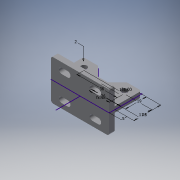
# Autodesk Inventor part: basepart
Saved by Autodesk Inventor 2018 (Build 220112000, 112)
## iProperties
Created: 2018-12-04
Part Number: basepart
Material: Generic
Document SubType Name: Modeling
Designer: Jerry
Density: 1 g/cm^3
Appearance: Default
Author: Jerry
Autodesk Inventor part; units mm, degrees
ref_plane "YZ Plane" through (0, 0, 0) normal (1, 0, 0) x (0, 1, 0)
ref_plane "XZ Plane" through (0, 0, 0) normal (0, 1, 0) x (-1, 0, 0)
ref_plane "XY Plane" through (0, 0, 0) normal (0, 0, 1) x (1, 0, 0)
sketch "Sketch1" plane through (0, 0, 0) normal (0, 0, 1) x (1, 0, 0)
  line L0 (0, 0) -> (0, -31.9527)
  line L1 (13.6569, 19) -> (24, 19)
  line L2 (1.4142, 7.5858) -> (12.2426, 18.4142)
  line L3 (26, 17) -> (26, -10)
  line L4 (26, -10) -> (0, -10)
  line L5 (-13.6569, 19) -> (-24, 19)
  line L6 (-1.4142, 7.5858) -> (-12.2426, 18.4142)
  line L7 (-26, 17) -> (-26, -10)
  line L8 (-26, -10) -> (0, -10)
  line L9 (-26, -5) -> (26, -5)
  arc A0 (-24, 19) -> (-26, 17) centre (-24, 17) ccw
  arc A1 (-12.2426, 18.4142) -> (-13.6569, 19) centre (-13.6569, 17) ccw
  arc A2 (-1.4142, 7.5858) -> (1.4142, 7.5858) centre (0, 9) ccw
  arc A3 (13.6569, 19) -> (12.2426, 18.4142) centre (13.6569, 17) ccw
  arc A4 (26, 17) -> (24, 19) centre (24, 17) ccw
  point P0 (-18, 11.5)
  point P1 (18, 11.5)
  point P2 (12.8284, 19)
  point P3 (26, 19)
  point P4 (-12.8284, 19)
  point P5 (-26, 19)
  dimension "d0" = 36
  dimension "d1" = 18
  dimension "d2" = 135
  dimension "d3" = 19
  dimension "d4" = 11.5
  dimension "d5" = 5
  dimension "d6" = 24
  dimension "d7" = 26
  dimension "d10" = 2
  dimension "d11" = 10
  constraints: 20 end point, 11 point on line, 10 point on circle, 10 tangent, 5 centre point, 4 equal radius, 3 symmetric about line, 2 perpendicular, 2 vertical, 1 horizontal, 1 horizontal alignment, 1 vertical alignment
  measures "d0" distance of point (-18, 11.5) point (18, 11.5)
  measures "d1" horizontal distance of L0.start point (18, 11.5)
  measures "d2" angle of L1 L2
  measures "d3" distance from line of L0.start L1
  measures "d4" vertical distance of L0.start point (-18, 11.5)
  measures "d5" distance between parallel lines of L4 L9
  measures "d6" distance between parallel lines of L1 L9
  measures "d7" distance from line of L0.start L3
  measures "d10" radius of A0
  measures "d11" distance from line of L1 A2.centre
extrude "Extrusion1" add sketch "Sketch1" along normal mid plane 5 contours L9 L7 A0 L5 A1 L6 A2 L2 A3 L1 A4 L3
hole "Hole1" at (-18, 11.5, 0) at (18, 11.5, 0) direction (0, 0, -1) diameter 5.159 end through all both
extrude "Extrusion2" add sketch "Sketch1" along normal mid plane 36 contours L9 L3 L4 L0 | L0 L8 L7 L9
fillet "Fillet1" radius 2 4 edges at (-26, -7.5, 18) (26, -7.5, 18) (-26, -7.5, -18) (26, -7.5, -18)
sketch "Sketch2" plane through (-26, -5, -2.5) normal (0, 1, 0) x (1, 0, 0)
  line L0 (42.418, 8.7532) -> (37.087, 8.7532) construction
  line L1 (42.418, 11.2532) -> (37.087, 11.2532)
  line L2 (37.087, 6.2532) -> (42.418, 6.2532)
  arc A0 (42.418, 6.2532) -> (42.418, 11.2532) centre (42.418, 8.7532) ccw
  arc A1 (37.087, 11.2532) -> (37.087, 6.2532) centre (37.087, 8.7532) ccw
  line L3 (69.9256, -2.5) -> (59.9264, -2.5) projected
  line L4 (36.6897, -2.5) -> (64.1036, -2.5) projected
  line L5 (42.418, -13.7532) -> (37.087, -13.7532) construction
  line L6 (42.418, -16.2532) -> (37.087, -16.2532)
  line L7 (37.087, -11.2532) -> (42.418, -11.2532)
  arc A2 (42.418, -16.2532) -> (42.418, -11.2532) centre (42.418, -13.7532) ccw
  arc A3 (37.087, -11.2532) -> (37.087, -16.2532) centre (37.087, -13.7532) ccw
  line L8 (52, 0) -> (0, 0) projected
  line L9 (26, 0) -> (26, 17.4848)
  line L10 (9.582, 8.7532) -> (14.913, 8.7532) construction
  line L11 (9.582, 11.2532) -> (14.913, 11.2532)
  line L12 (14.913, 6.2532) -> (9.582, 6.2532)
  arc A4 (9.582, 11.2532) -> (9.582, 6.2532) centre (9.582, 8.7532) ccw
  arc A5 (14.913, 6.2532) -> (14.913, 11.2532) centre (14.913, 8.7532) ccw
  line L13 (9.582, -13.7532) -> (14.913, -13.7532) construction
  line L14 (9.582, -16.2532) -> (14.913, -16.2532)
  line L15 (14.913, -11.2532) -> (9.582, -11.2532)
  arc A6 (9.582, -11.2532) -> (9.582, -16.2532) centre (9.582, -13.7532) ccw
  arc A7 (14.913, -16.2532) -> (14.913, -11.2532) centre (14.913, -13.7532) ccw
  point P0 (26, -2.5)
  point P1 (39.7525, 8.7532)
  point P2 (39.7525, -13.7532)
  point P3 (26, -2.5)
  point P4 (26, -2.5)
  point P5 (26, -2.5)
  point P6 (12.2475, 8.7532)
  point P7 (15.3103, -2.5)
  point P8 (12.2475, -13.7532)
  dimension "d24" = 5
  constraints: 34 end point, 22 symmetric about line, 16 point on circle, 8 centre point, 4 tangent, 2 midpoint, 1 horizontal, 1 parallel, 1 vertical, 6 other
  measures "d24" diameter of A1
extrude "Extrusion3" cut sketch "Sketch2" against normal through all
equation "\"d1\" = 0.5 * d0"
body "Solid1"
